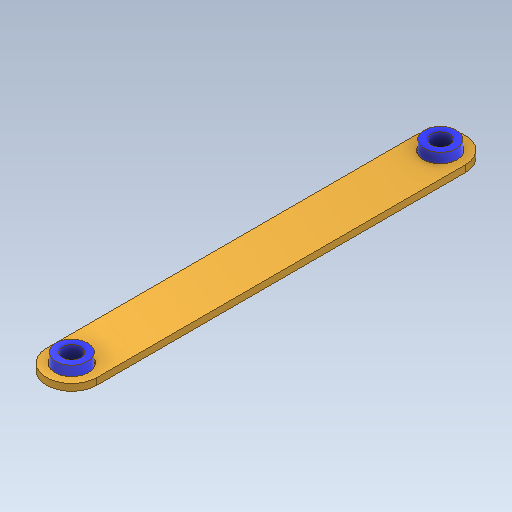
# Autodesk Inventor part: connecting rod
Saved by Autodesk Inventor 2020 (Build 240168000, 168)
## iProperties
Created: 2020-07-28
Part Number: connecting rod
Material: Steel, Mild
Document SubType Name: Modeling
Designer: Vikki
Density: 7.85 g/cm^3
Appearance: Brass - Satin
Mass: 1907.51 g
Surface Area: 729.46 cm^2
Volume: 242.995 cm^3
Author: Vikki
Autodesk Inventor part; units mm, degrees
ref_plane "YZ Plane" through (0, 0, 0) normal (1, 0, 0) x (0, 1, 0)
ref_plane "XZ Plane" through (0, 0, 0) normal (0, 1, 0) x (-1, 0, 0)
sketch "Sketch1" plane through (0, 0, 0) normal (0, 1, 0) x (-1, 0, 0)
  circle A0 centre (0, 0) radius 10
  line L0 (0, 0) -> (0, -437.5) construction
  line L1 (-30, 0) -> (-30, -437.5)
  line L2 (30, -437.5) -> (30, 0)
  arc A1 (30, 0) -> (-30, 0) centre (0, 0) ccw
  arc A2 (-30, -437.5) -> (30, -437.5) centre (0, -437.5) ccw
  circle A3 centre (0, -437.5) radius 10
  point P0 (0, -218.75)
  dimension "d0" = 20
  dimension "d1" = 437.5
  dimension "d2" = 20
  dimension "d3" = 30
  constraints: 8 end point, 4 centre point, 4 point on circle, 4 tangent, 2 coincident, 1 midpoint, 1 parallel, 1 vertical
  measures "d0" diameter of A0
  measures "d1" distance of point (0, 0) L0.end
  measures "d2" diameter of A3
  measures "d3" radius of A2
extrude "Extrusion1" add sketch "Sketch1" along normal blind 8
sketch "Sketch2" plane through (0, 8, 0) normal (0, 1, 0) x (1, 0, 0)
  circle A0 centre (0, 0) radius 20
  circle A1 centre (0, 437.5) radius 10 projected
  circle A2 centre (0, 437.5) radius 10 projected
  circle A3 centre (0, 437.5) radius 20
  circle A4 centre (0, 0) radius 10 projected
  dimension "d6" = 40
  constraints: 2 centre point, 2 coincident, 1 equal radius
  measures "d6" diameter of A0
extrude "Extrusion2" cut sketch "Sketch2" against normal blind 4
sketch "Sketch3" plane through (0, 0, 0) normal (0, -1, 0) x (1, 0, 0)
  circle A0 centre (0, 0) radius 9 projected
  circle A1 centre (0, 0) radius 11.5
  point P0 (0, 0)
  dimension "d9" = 23
  constraints: 1 centre point, 1 coincident
  measures "d9" diameter of A1
extrude "Extrusion3" add sketch "Sketch3" along normal blind 2
sketch "Sketch4" plane through (0, 4, 0) normal (0, 1, 0) x (1, 0, 0)
  circle A0 centre (0, 0) radius 20 projected
  circle A1 centre (0, 0) radius 10 projected
  circle A2 centre (0, 437.5) radius 20 projected
  circle A3 centre (0, 437.5) radius 10 projected
  circle A4 centre (0, 0) radius 19
  circle A5 centre (0, 0) radius 11
  dimension "d12" = 38
  dimension "d13" = 22
  constraints: 2 centre point, 2 coincident
  measures "d12" diameter of A4
  measures "d13" diameter of A5
extrude "Extrusion4" add sketch "Sketch4" along normal blind 15 contours A4
ref_plane "Work Plane1" through (0, 0, -218.75) normal (0, 0, 1) x (1, 0, 0)
mirror "Mirror1" about plane through (0, 0, -218.75) normal (0, 0, 1) of "Extrusion4"
body "Solid1"
